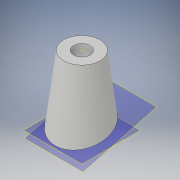
# Autodesk Inventor part: cone
Saved by Autodesk Inventor 2019 (Build 230136000, 136)
## iProperties
Created: 2020-10-26
Part Number: cone
Material: Genérico
Document SubType Name: Modeling
Designer: Juan M. Casillas
Density: 1 g/cm^3
Appearance: Valor por defecto
Author: Juan M. Casillas
Autodesk Inventor part; units mm, degrees
ref_plane "YZ Plane" through (0, 0, 0) normal (1, 0, 0) x (0, 1, 0)
ref_plane "XZ Plane" through (0, 0, 0) normal (0, 1, 0) x (-1, 0, 0)
ref_plane "XY Plane" through (0, 0, 0) normal (0, 0, 1) x (1, 0, 0)
sketch "Sketch1" plane through (0, 0, 0) normal (0, 1, 0) x (-1, 0, 0)
  circle A0 centre (0, 0) radius 10
  circle A1 centre (0, 0) radius 3.1
  dimension "d0" = 20
  dimension "d1" = 6.2
  constraints: 2 centre point, 2 coincident
  measures "d0" diameter of A0
  measures "d1" diameter of A1
extrude "Extrusion1" add sketch "Sketch1" along normal blind 26
ref_plane "Work Plane3" through (0, 2.5114, 0.6729) normal (0, -0.9659258, -0.258819) x (1, 0, 0)
ref_plane "Work Plane2" through (0, 0, 0) normal (0, -0.9659258, -0.258819) x (1, 0, 0)
draft "FaceDraft1" angle 7 pull direction (0, 1, 0) faces at (-9.8705, 17.3333, -1.6041) fixed edges at (10, 0, 0)
sketch "Sketch2" plane through (0, 26, 0) normal (0, 1, 0) x (1, 0, 0)
  point P0 (0, 0)
split "Split1" plane through (0, 2.5114, 0.6729) removes the side toward (0, -0.9659258, -0.258819)
ref_plane "Work Plane1" through (0, 0, 0) normal (0, -1, 0) x (1, 0, 0)
body "Solid1"
